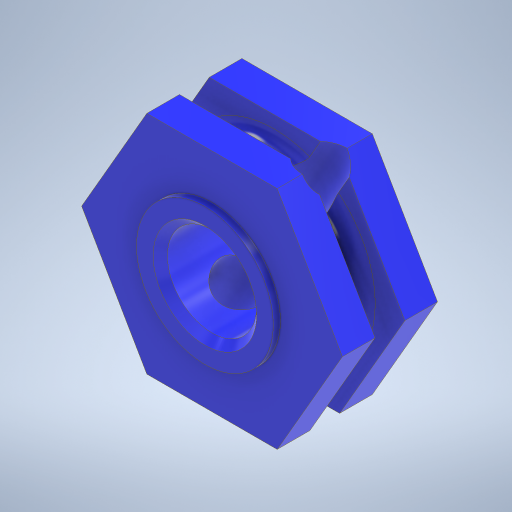
# Autodesk Inventor part: HexDrive
Saved by Autodesk Inventor 2024 (Build 280153000, 153)
## iProperties
Created: 2023-05-27
Part Number: HexDrive
Material: Nylon 6/6
Document SubType Name: Modeling
Designer: _Astitva_Aryan_
Density: 1.13 g/cm^3
Appearance: Nylon 6
Author: _Astitva_Aryan_
Autodesk Inventor part; units mm, degrees
ref_plane "YZ Plane" through (0, 0, 0) normal (1, 0, 0) x (0, 1, 0)
ref_plane "XZ Plane" through (0, 0, 0) normal (0, 1, 0) x (-1, 0, 0)
ref_plane "XY Plane" through (0, 0, 0) normal (0, 0, 1) x (1, 0, 0)
sketch "Sketch1" plane through (0, 0, 0) normal (0, 0, 1) x (1, 0, 0)
  circle A0 centre (0, 0) radius 6.0325 construction
  line L0 (3.4829, 6.0325) -> (6.9657, 0)
  line L1 (6.9657, 0) -> (3.4829, -6.0325)
  line L2 (3.4829, -6.0325) -> (-3.4829, -6.0325)
  line L3 (-3.4829, -6.0325) -> (-6.9657, 0)
  line L4 (-6.9657, 0) -> (-3.4829, 6.0325)
  line L5 (-3.4829, 6.0325) -> (3.4829, 6.0325)
  point P0 (0, 6.0325)
  dimension "d0" = 12.065
  constraints: 12 end point, 2 coincident, 1 horizontal, 1 midpoint, 1 vertical alignment, 15 other
extrude "Extrusion1" add sketch "Sketch1" along normal mid plane 5.08
sketch "Sketch2" plane through (0, 0, 2.54) normal (0, 0, 1) x (1, 0, 0)
  circle A0 centre (0, 0) radius 2.3813
  circle A1 centre (0, 0) radius 3.6513
  dimension "d3" = 4.7625
  dimension "d4" = 1.27
  constraints: 2 centre point, 1 coincident
  measures "d3" diameter of A0
  measures "d4" radial gap between concentric circles of A0 A1
extrude "Extrusion2" cut sketch "Sketch2" against normal blind 5.08 contours A0
extrude "Extrusion3" add sketch "Sketch2" along normal blind 0.381
chamfer "Chamfer1" distance 0.381 angle 45 1 edges at (-2.3813, 0, 2.921)
ref_plane "Work Plane1" through (3.4829, 6.0325, 0) normal (0.5, 0.8660254, 0) x (0, 0, 1)
sketch "Sketch3" plane through (3.4829, 6.0325, 0) normal (0.5, 0.8660254, 0) x (0, 0, 1)
  circle A0 centre (0, 0) radius 1.1913
  dimension "d13" = 2.3825
  constraints: 1 centre point, 1 coincident
  measures "d13" diameter of A0
extrude "Extrusion4" cut sketch "Sketch3" against normal through all
ref_plane "Work Plane3" through (3.4829, 6.0325, 0) normal (0.8660254, -0.5, 0) x (0, 0, 1)
sketch "Sketch7" plane through (3.4829, 6.0325, 0) normal (0.8660254, -0.5, 0) x (0, 0, 1)
  line L0 (-0.7937, 0) -> (-0.7937, 1.5875)
  arc A0 (0.7937, 1.5875) -> (-0.7937, 1.5875) centre (0, 1.5875) ccw
  line L1 (0.7937, 1.5875) -> (0.7938, 0)
  line L2 (-0.7937, 0) -> (0.7938, 0)
  line L3 (2.54, 3.4829) -> (2.54, 0) projected
  line L4 (2.54, 0) -> (1.1913, 0)
  line L5 (1.1913, 0) -> (1.1913, 4.5845) projected
  line L6 (-3.6322, 6.9657) -> (4.0132, 6.9657) projected
  point P0 (0, 6.9657)
  dimension "d16" = 1.5875
  dimension "d17" = 1.5875
  constraints: 8 end point, 2 point on circle, 2 vertical, 1 centre point, 1 collinear, 1 horizontal, 1 perpendicular, 1 point on line, 1 tangent, 1 vertical alignment
  measures "d16" distance of L0.start L0.end
  measures "d17" diameter of A0
revolve "Revolution1" cut sketch "Sketch7" angle 360 about axis through (0, 0, -10) along (0, 0, 1)
scale "Scale1" factors (10, 10, 10) then translate (0, 0, 22.86) bodies 1
body "Solid1"
